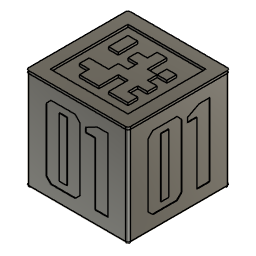
AutonOhm Apriltag 01 (Autodesk Fusion 360 design; units mm, degrees)
Autodesk Fusion 360 part; units mm, degrees
sketch "Skizze1" plane through (0, 0, 0) normal (0, 0, 1) x (1, 0, 0)
  line L0 (21, -21) -> (-21, -21)
  line L1 (-21, -21) -> (-21, 21)
  line L2 (-21, 21) -> (21, 21)
  line L3 (21, 21) -> (21, -21)
  line L4 (21, -21) -> (-21, 21) construction
  line L5 (-21, -21) -> (21, 21) construction
  dimension "d1" = 42
  dimension "d2" = 42
  constraint horizontal L0
  constraint perpendicular L0 L1
  constraint parallel L0 L2
  constraint parallel L1 L3
  constraint coincident L4 origin
  constraint coincident L5 origin
  measures "d1" distance of L1.end L2.end
  measures "d2" distance of L0.end L1.end
extrude "Extrusion1" add sketch "Skizze1" along normal blind 41 makes body 1
sketch "Skizze2" plane through (0, 0, 41) normal (0, 0, 1) x (-1, 0, 0)
  line L0 (-21, -21) -> (21, -21)
  line L1 (21, -21) -> (21, 21)
  line L2 (21, 21) -> (-21, 21)
  line L3 (-21, 21) -> (-21, -21)
  line L4 (21, -21) -> (-21, -21)
  line L5 (-21, -21) -> (-21, 21)
  line L6 (-21, 21) -> (21, 21)
  line L7 (21, 21) -> (21, -21)
  line L8 (-16, 16) -> (16, 16)
  line L9 (16, 16) -> (16, -16)
  line L10 (16, -16) -> (-16, -16)
  line L11 (-16, -16) -> (-16, 16)
  line L12 (-16, 16) -> (16, -16) construction
  line L13 (16, 16) -> (-16, -16) construction
  dimension "d5" = 32
  dimension "d6" = 32
  constraint horizontal L4
  constraint vertical L5
  constraint horizontal L6
  constraint vertical L7
  constraint coincident L2.end L3.start
  constraint coincident L0.end L1.start
  constraint horizontal L8
  constraint perpendicular L8 L9
  constraint parallel L8 L10
  constraint parallel L9 L11
  constraint coincident L12 origin
  constraint coincident L13 origin
  measures "d5" distance of L9.end L10.end
  measures "d6" distance of L8.end L9.end
extrude "Extrusion2" add sketch "Skizze2" along normal blind 1 separate body makes body 2
fillet "Abrundung1" radius 1 8 edges at (-21, 21, 20.5) (-21, -21, 20.5) (-21, 0, 0) (0, -21, 0) (21, -21, 20.5) (21, 0, 0) (21, 21, 20.5) (0, 21, 0) on bodies 1
fillet "Abrundung2" radius 1 1 edges at (21, 21, 41.5) on bodies 2
fillet "Abrundung3" radius 1 1 edges at (21, -21, 41.5) on bodies 2
fillet "Abrundung4" radius 1 1 edges at (-21, -21, 41.5) on bodies 2
fillet "Abrundung5" radius 1 1 edges at (-21, 21, 41.5) on bodies 2
sketch "Skizze3" plane through (0, 0, 0) normal (0, 0, -1) x (1, 0, 0)
  line L0 (-20, -20) -> (20, -20)
  line L1 (20, -20) -> (20, 20)
  line L2 (20, 20) -> (-20, 20)
  line L3 (-20, 20) -> (-20, -20)
  line L4 (-15.5554, -7.5319) -> (-15.5554, -12.9394)
  line L5 (-15.5554, -12.9394) -> (-1.7653, -13.0619)
  line L6 (-1.7653, -13.0619) -> (-1.8353, -7.8468)
  spline S0 degree 3 poles (-1.8353, -7.8468) (-9.4573, -5.9337) (-9.4543, 8.1703) (-0.2245, 8.2733) knots 0 0 0 0 1 1 1 1
  spline S1 degree 3 poles (-0.2245, 8.2733) (9.1628, 8.378) (10.5465, -5.8261) (1.9583, -7.8813) knots 0 0 0 0 1 1 1 1
  line L7 (1.9583, -7.8813) -> (1.9723, -13.0334)
  spline S2 degree 3 poles (1.9723, -13.0334) (15.5516, -12.9722) (18.9797, 12.8679) (-0.1523, 13.061) knots 0 0 0 0 1 1 1 1
  spline S3 degree 3 poles (-0.1523, 13.061) (-11.1806, 13.1724) (-15.9327, 2.2058) (-10.2013, -7.6521) knots 0 0 0 0 1 1 1 1
  line L8 (-10.2013, -7.6521) -> (-15.5554, -7.5319)
extrude "Extrusion3" add sketch "Skizze3" against normal blind 0.6 separate body contours L4 L5 L6 S0 S1 L7 S2 S3 L8 makes body 3
sketch "Skizze4" plane through (0, 0, 41) normal (0, 0, 1) x (-1, 0, 0)
  arc A0 (21, 20) -> (20, 21) centre (20, 20) ccw
  line L0 (20, 21) -> (-20, 21)
  arc A1 (-20, 21) -> (-21, 20) centre (-20, 20) ccw
  line L1 (-21, 20) -> (-21, -20)
  arc A2 (-21, -20) -> (-20, -21) centre (-20, -20) ccw
  line L2 (-20, -21) -> (20, -21)
  arc A3 (20, -21) -> (21, -20) centre (20, -20) ccw
  line L3 (21, -20) -> (21, 20)
  line L4 (-20, 20) -> (20, 20)
  line L5 (20, 20) -> (20, -20)
  line L6 (20, -20) -> (-20, -20)
  line L7 (-20, -20) -> (-20, 20)
  line L8 (-15.9999, 15.9999) -> (16.0002, 15.9999)
  line L9 (16.0002, 15.9999) -> (16.0002, -16.0002)
  line L10 (16.0002, -16.0002) -> (-15.9999, -16.0002)
  line L11 (-15.9999, -16.0002) -> (-15.9999, 15.9999)
  line L12 (-12.0001, 12.0001) -> (-12.0001, 7.9999)
  line L13 (-12.0001, 7.9999) -> (-7.9999, 7.9999)
  line L14 (-7.9999, 7.9999) -> (-7.9999, 4.0002)
  line L15 (-7.9999, 4.0002) -> (-12.0001, 4.0002)
  line L16 (-12.0001, 4.0002) -> (-12.0001, 0)
  line L17 (-12.0001, 0) -> (-7.9999, 0)
  line L18 (-7.9999, 0) -> (-7.9999, -3.9998)
  line L19 (-7.9999, -3.9998) -> (-12.0001, -3.9998)
  line L20 (-12.0001, -3.9998) -> (-12.0001, -7.9999)
  line L21 (-12.0001, -7.9999) -> (-7.9999, -7.9999)
  line L22 (-7.9999, -7.9999) -> (-7.9999, -3.9998)
  line L23 (-7.9999, -3.9998) -> (-4.0002, -3.9998)
  line L24 (-4.0002, -3.9998) -> (-4.0002, -12)
  line L25 (-4.0002, -12) -> (0, -12)
  line L26 (0, -12) -> (0, -7.9999)
  line L27 (0, -7.9999) -> (3.9998, -7.9999)
  line L28 (3.9998, -7.9999) -> (3.9998, -3.9998)
  line L29 (3.9998, -3.9998) -> (0, -3.9998)
  line L30 (0, -3.9998) -> (0, 0)
  line L31 (0, 0) -> (3.9998, 0)
  line L32 (3.9998, 0) -> (3.9998, 4.0002)
  line L33 (3.9998, 4.0002) -> (12, 4.0002)
  line L34 (12, 4.0002) -> (12, 7.9999)
  line L35 (12, 7.9999) -> (7.9999, 7.9999)
  line L36 (7.9999, 7.9999) -> (7.9999, 12.0001)
  line L37 (7.9999, 12.0001) -> (0, 12.0001)
  line L38 (0, 12.0001) -> (0, 4.0002)
  line L39 (0, 4.0002) -> (-4.0002, 4.0002)
  line L40 (-4.0002, 4.0002) -> (-4.0002, 12.0001)
  line L41 (-4.0002, 12.0001) -> (-12.0001, 12.0001)
  line L42 (7.9999, -3.9998) -> (7.9999, -12)
  line L43 (7.9999, -12) -> (12, -12)
  line L44 (12, -12) -> (12, -3.9998)
  line L45 (12, -3.9998) -> (7.9999, -3.9998)
extrude "Extrusion4" add sketch "Skizze4" along normal blind 1 separate body contours L12 L13 L14 L15 L16 L17 L18 L23 L24 L25 L26 L27 L28 L29 L30 L31 L32 L33 L34 L35 L36 L37 L38 L39 L40 L41 | L19 L20 L21 L22 | L42 L43 L44 L45 makes body 4 at (-3.9999, -8.0001, 41) makes body 4 at (9.3333, 5.3331, 41) makes body 5 at (-9.3333, 6.6665, 41)
sketch "Skizze5" plane through (0, 21, 0) normal (0, 1, 0) x (-1, 0, 0)
  line L0 (20, 1) -> (20, 41)
  line L1 (20, 41) -> (-20, 41)
  line L2 (-20, 41) -> (-20, 1)
  line L3 (-20, 1) -> (20, 1)
  line L4 (1.1893, 33.9386) -> (-0.7634, 35.9978)
  line L5 (-0.7634, 35.9978) -> (-10.7752, 35.9978)
  line L6 (-10.7752, 35.9978) -> (-12.7278, 33.9386)
  line L7 (-12.7278, 33.9386) -> (-12.7278, 7.9505)
  line L8 (-12.7278, 7.9505) -> (-10.7752, 5.9979)
  line L9 (-10.7752, 5.9979) -> (-0.7634, 5.9979)
  line L10 (-0.7634, 5.9979) -> (1.1893, 7.9505)
  line L11 (1.1893, 7.9505) -> (1.1893, 33.9386)
  line L12 (-7.3669, 8.8381) -> (-7.3669, 33.1575)
  line L13 (-7.3669, 33.1575) -> (-4.1716, 33.1575)
  line L14 (-4.1716, 33.1575) -> (-4.1716, 8.8381)
  line L15 (-4.1716, 8.8381) -> (-7.3669, 8.8381)
  line L16 (12.7277, 35.9978) -> (8.3254, 35.9978)
  line L17 (8.3254, 35.9978) -> (3.5325, 33.5126)
  line L18 (3.5325, 33.5126) -> (3.5325, 31.6309)
  line L19 (3.5325, 31.6309) -> (7.4023, 31.6309)
  line L20 (7.4023, 31.6309) -> (7.4023, 5.9979)
  line L21 (7.4023, 5.9979) -> (12.7277, 5.9979)
  line L22 (12.7277, 5.9979) -> (12.7277, 35.9978)
extrude "Extrusion5" cut sketch "Skizze5" against normal blind 0.2 contours L4 L5 L6 L7 L8 L9 L10 L11 | L16 L17 L18 L19 L20 L21 L22 bodies 1
sketch "Skizze6" plane through (21, 0, 0) normal (1, 0, 0) x (0, 1, 0)
  line L0 (-20, 41) -> (-20, 1)
  line L1 (-20, 1) -> (20, 1)
  line L2 (20, 1) -> (20, 41)
  line L3 (20, 41) -> (-20, 41)
  line L4 (1.1893, 33.9386) -> (-0.7634, 35.9978)
  line L5 (-0.7634, 35.9978) -> (-10.7752, 35.9978)
  line L6 (-10.7752, 35.9978) -> (-12.7278, 33.9386)
  line L7 (-12.7278, 33.9386) -> (-12.7278, 7.9505)
  line L8 (-12.7278, 7.9505) -> (-10.7752, 5.9979)
  line L9 (-10.7752, 5.9979) -> (-0.7634, 5.9979)
  line L10 (-0.7634, 5.9979) -> (1.1893, 7.9505)
  line L11 (1.1893, 7.9505) -> (1.1893, 33.9386)
  line L12 (-7.3669, 8.8381) -> (-7.3669, 33.1575)
  line L13 (-7.3669, 33.1575) -> (-4.1716, 33.1575)
  line L14 (-4.1716, 33.1575) -> (-4.1716, 8.8381)
  line L15 (-4.1716, 8.8381) -> (-7.3669, 8.8381)
  line L16 (12.7277, 35.9978) -> (8.3254, 35.9978)
  line L17 (8.3254, 35.9978) -> (3.5325, 33.5126)
  line L18 (3.5325, 33.5126) -> (3.5325, 31.6309)
  line L19 (3.5325, 31.6309) -> (7.4023, 31.6309)
  line L20 (7.4023, 31.6309) -> (7.4023, 5.9979)
  line L21 (7.4023, 5.9979) -> (12.7277, 5.9979)
  line L22 (12.7277, 5.9979) -> (12.7277, 35.9978)
extrude "Extrusion6" cut sketch "Skizze6" against normal blind 0.2 contours L4 L5 L6 L7 L8 L9 L10 L11 | L16 L17 L18 L19 L20 L21 L22 bodies 1
sketch "Skizze7" plane through (0, -21, 0) normal (0, -1, 0) x (1, 0, 0)
  line L0 (-20, 41) -> (-20, 1)
  line L1 (-20, 1) -> (20, 1)
  line L2 (20, 1) -> (20, 41)
  line L3 (20, 41) -> (-20, 41)
  line L4 (1.1893, 33.9386) -> (-0.7634, 35.9978)
  line L5 (-0.7634, 35.9978) -> (-10.7752, 35.9978)
  line L6 (-10.7752, 35.9978) -> (-12.7278, 33.9386)
  line L7 (-12.7278, 33.9386) -> (-12.7278, 7.9505)
  line L8 (-12.7278, 7.9505) -> (-10.7752, 5.9979)
  line L9 (-10.7752, 5.9979) -> (-0.7634, 5.9979)
  line L10 (-0.7634, 5.9979) -> (1.1893, 7.9505)
  line L11 (1.1893, 7.9505) -> (1.1893, 33.9386)
  line L12 (-7.3669, 8.8381) -> (-7.3669, 33.1575)
  line L13 (-7.3669, 33.1575) -> (-4.1716, 33.1575)
  line L14 (-4.1716, 33.1575) -> (-4.1716, 8.8381)
  line L15 (-4.1716, 8.8381) -> (-7.3669, 8.8381)
  line L16 (12.7277, 35.9978) -> (8.3254, 35.9978)
  line L17 (8.3254, 35.9978) -> (3.5325, 33.5126)
  line L18 (3.5325, 33.5126) -> (3.5325, 31.6309)
  line L19 (3.5325, 31.6309) -> (7.4023, 31.6309)
  line L20 (7.4023, 31.6309) -> (7.4023, 5.9979)
  line L21 (7.4023, 5.9979) -> (12.7277, 5.9979)
  line L22 (12.7277, 5.9979) -> (12.7277, 35.9978)
extrude "Extrusion7" cut sketch "Skizze7" against normal blind 0.2 contours L4 L5 L6 L7 L8 L9 L10 L11 | L16 L17 L18 L19 L20 L21 L22 bodies 1
sketch "Skizze8" plane through (-21, 0, 0) normal (-1, 0, 0) x (0, -1, 0)
  line L0 (20, 1) -> (20, 41)
  line L1 (20, 41) -> (-20, 41)
  line L2 (-20, 41) -> (-20, 1)
  line L3 (-20, 1) -> (20, 1)
  line L4 (1.1893, 33.9386) -> (-0.7634, 35.9978)
  line L5 (-0.7634, 35.9978) -> (-10.7752, 35.9978)
  line L6 (-10.7752, 35.9978) -> (-12.7278, 33.9386)
  line L7 (-12.7278, 33.9386) -> (-12.7278, 7.9505)
  line L8 (-12.7278, 7.9505) -> (-10.7752, 5.9979)
  line L9 (-10.7752, 5.9979) -> (-0.7634, 5.9979)
  line L10 (-0.7634, 5.9979) -> (1.1893, 7.9505)
  line L11 (1.1893, 7.9505) -> (1.1893, 33.9386)
  line L12 (-7.3669, 8.8381) -> (-7.3669, 33.1575)
  line L13 (-7.3669, 33.1575) -> (-4.1716, 33.1575)
  line L14 (-4.1716, 33.1575) -> (-4.1716, 8.8381)
  line L15 (-4.1716, 8.8381) -> (-7.3669, 8.8381)
  line L16 (12.7277, 35.9978) -> (8.3254, 35.9978)
  line L17 (8.3254, 35.9978) -> (3.5325, 33.5126)
  line L18 (3.5325, 33.5126) -> (3.5325, 31.6309)
  line L19 (3.5325, 31.6309) -> (7.4023, 31.6309)
  line L20 (7.4023, 31.6309) -> (7.4023, 5.9979)
  line L21 (7.4023, 5.9979) -> (12.7277, 5.9979)
  line L22 (12.7277, 5.9979) -> (12.7277, 35.9978)
extrude "Extrusion8" cut sketch "Skizze8" against normal blind 0.2 contours L4 L5 L6 L7 L8 L9 L10 L11 | L16 L17 L18 L19 L20 L21 L22 bodies 1
named bodies: "Grundkörper", "Apriltag Kranz", "OhmLogo Unterseite"
